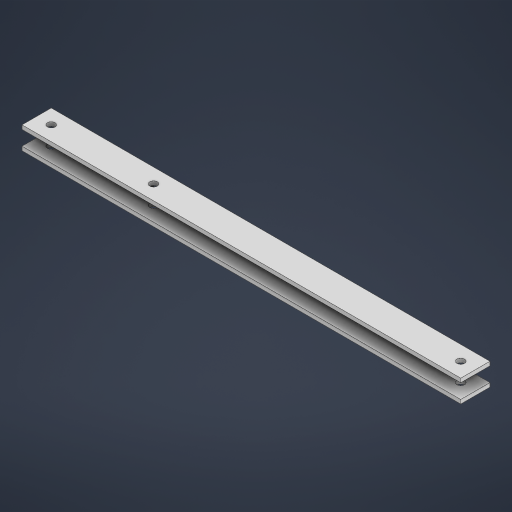
# Autodesk Inventor part: ArmPart3Mini
Saved by Autodesk Inventor 2024.2 (Build 282272000, 272)
## iProperties
Created: 2024-01-04
Part Number: ArmPart3Mini
Material: Generic
Document SubType Name: Modeling
Designer: student
Density: 1 g/cm^3
Appearance: Default
Author: student
Autodesk Inventor part; units mm, degrees
ref_plane "YZ Plane" through (0, 0, 0) normal (1, 0, 0) x (0, 1, 0)
ref_plane "XZ Plane" through (0, 0, 0) normal (0, 1, 0) x (-1, 0, 0)
ref_plane "XY Plane" through (0, 0, 0) normal (0, 0, 1) x (1, 0, 0)
sketch "Sketch1" plane through (0, 0, 0) normal (0, 1, 0) x (-1, 0, 0)
  line L0 (0, 0) -> (381, 0)
  line L1 (381, 0) -> (381, -25.4)
  line L2 (381, -25.4) -> (0, -25.4)
  line L3 (0, -25.4) -> (0, 0)
  dimension "d0" = 381
  dimension "d1" = 25.4
  constraints: 8 end point, 2 parallel, 1 horizontal, 1 perpendicular
  measures "d0" distance of L1.end L2.end
  measures "d1" distance of L0.end L1.end
extrude "Extrusion1" add sketch "Sketch1" along normal blind 3.429
sketch "Sketch2" plane through (0, 3.429, 0) normal (0, 1, 0) x (1, 0, 0)
  line L0 (0, 25.4) -> (-381, 25.4) projected
  line L1 (-38.1, 25.4) -> (-266.7, 25.4)
  line L2 (-266.7, 25.4) -> (-266.7, 21.7932)
  line L3 (-266.7, 21.7932) -> (-38.1, 21.7932)
  line L4 (-38.1, 21.7932) -> (-38.1, 25.4)
  line L5 (0, 0) -> (0, 25.4) projected
  line L6 (-292.1, 25.4) -> (-342.9, 25.4)
  line L7 (-342.9, 25.4) -> (-342.9, 21.7932)
  line L8 (-342.9, 21.7932) -> (-292.1, 21.7932)
  line L9 (-292.1, 21.7932) -> (-292.1, 25.4)
  point P0 (-266.7, 23.5966)
  dimension "d4" = 228.6
  dimension "d5" = 3.6068
  dimension "d6" = 38.1
  dimension "d7" = 50.8
  dimension "d8" = 3.6068
  dimension "d9" = 25.4
  constraints: 16 end point, 4 parallel, 2 horizontal, 2 perpendicular, 2 point on line, 1 midpoint
  measures "d4" distance of L3.end L2.end
  measures "d5" distance of L2.end L1.end
  measures "d6" distance between parallel lines of L5 L4
  measures "d7" distance of L8.end L7.end
  measures "d8" distance of L8.end L6.start
  measures "d9" distance from line of point (-266.7, 23.597) L9
extrude "Extrusion2" add sketch "Sketch2" along normal blind 12.5984
sketch "Sketch3" plane through (0, 16.0274, 0) normal (0, 1, 0) x (1, 0, 0)
  line L0 (-381, 0) -> (0, 0) projected
  line L1 (0, 25.4) -> (-381, 25.4) projected
  line L2 (-381, 0) -> (0, 0)
  line L3 (0, 0) -> (0, 25.4)
  line L4 (0, 25.4) -> (-381, 25.4)
  line L5 (-381, 25.4) -> (-381, 0)
  constraints: 8 end point, 2 parallel, 1 horizontal, 1 perpendicular
extrude "Extrusion3" add sketch "Sketch3" along normal blind 3.429
sketch "Sketch4" plane through (0, 19.4564, 0) normal (0, 1, 0) x (1, 0, 0)
  line L0 (0, 25.4) -> (-381, 25.4) projected
  line L1 (0, 0) -> (0, 25.4) projected
  point P0 (-12.7, 12.7)
  dimension "d14" = 12.7
  dimension "d15" = 12.7
  measures "d14" distance from line of L0 point (-12.7, 12.7)
  measures "d15" distance from line of L1 point (-12.7, 12.7)
hole "Hole1" at (-12.7, 19.4564, -12.7) direction (0, -1, 0) diameter 6.5024 end through all
sketch "Sketch5" plane through (0, 19.4564, 0) normal (0, 1, 0) x (1, 0, 0)
  line L0 (0, 25.4) -> (-381, 25.4) projected
  line L1 (-381, 25.4) -> (-381, 0) projected
  point P0 (0, 0)
  point P1 (-279.4, 12.7)
  point P2 (-381, 12.7)
  dimension "d23" = 12.7
  dimension "d40" = 101.6
  constraints: 1 midpoint
  measures "d23" distance from line of L0 point (-279.4, 12.7)
  measures "d40" distance of point (-381, 12.7) point (-279.4, 12.7)
hole "Hole2" at (-279.4, 19.4564, -12.7) direction (0, -1, 0) diameter 6.5024 end through all
sketch "Sketch6" plane through (0, 19.4564, 0) normal (0, 1, 0) x (1, 0, 0)
  line L0 (0, 25.4) -> (-381, 25.4) projected
  line L1 (-381, 25.4) -> (-381, 0) projected
  point P0 (0, 0)
  point P1 (-368.3, 12.7)
  dimension "d31" = 12.7
  dimension "d32" = 12.7
  measures "d31" distance from line of L0 point (-368.3, 12.7)
  measures "d32" distance from line of L1 point (-368.3, 12.7)
hole "Hole3" at (-368.3, 19.4564, -12.7) direction (0, -1, 0) diameter 6.5024 end through all
body "Solid1"
